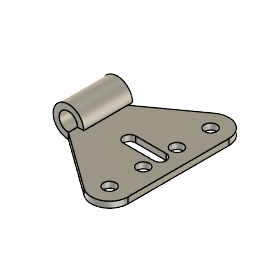
50 (Autodesk Fusion 360 design; units mm, degrees)
Autodesk Fusion 360 part; units mm, degrees
sketch "草图1" plane through (0, 0, 0) normal (0, 1, 0) x (1, 0, 0)
  line L0 (28, 3) -> (28, 5)
  line L1 (28, 5) -> (0, 5)
  arc A0 (0, 5) -> (5, 0) centre (0, 0) ccw
  line L2 (28, 3) -> (0, 3)
  arc A1 (0, 3) -> (3, 0) centre (0, 0) ccw
  line L3 (3, 0) -> (5, 0)
  line L4 (0, 3) -> (0, 5)
  dimension "d1" = 2
  dimension "d2" = 3
  dimension "d3" = 5
  dimension "d4" = 2
  dimension "d5" = 28
  constraint vertical L0
  constraint perpendicular L0 L1
  constraint tangent L1 A0
  constraint perpendicular L0 L2
  constraint tangent L2 A1
  constraint parallel L2 L3
  constraint coincident A0.centre A1.centre
  measures "d1" distance of L0.start L0.end
  measures "d2" radius of A1
  measures "d3" radius of A0
  measures "d4" distance of A0.end A1.end
  measures "d5" distance of L0.end L1.end
extrude "拉伸1" add sketch "草图1" along normal mid plane 16 contours A0 A1 L3 L4
extrude "拉伸2" add sketch "草图1" along normal mid plane 45 contours L0 L1 L2 L4
sketch "草图2" plane through (0, 0, -3) normal (0, 0, 1) x (-1, 0, 0)
  line L0 (-28, 22.5) -> (-28, -22.5)
  line L1 (-28, -22.5) -> (0, -22.5)
  line L2 (0, -22.5) -> (0, -8)
  line L3 (0, -8) -> (0, 8)
  line L4 (0, 8) -> (0, 22.5)
  line L5 (0, 22.5) -> (-28, 22.5)
  line L6 (0, -8) -> (-18.4849, -21.3625)
  arc A0 (-28, -16.5) -> (-18.4849, -21.3625) centre (-22, -16.5) ccw
  line L7 (-28, -16.5) -> (-28, 16.5)
  arc A1 (-18.4849, 21.3625) -> (-28, 16.5) centre (-22, 16.5) ccw
  line L8 (-18.4849, 21.3625) -> (0, 8)
  line L9 (0, 8) -> (0, -8)
  line L10 (10, 0) -> (-55, 0) construction
  circle A2 centre (-22, -16.5) radius 2
  circle A3 centre (-22, 16.5) radius 2
  line L11 (-22, -16.5) -> (-22, 16.5) construction
  circle A4 centre (-22, -5.5) radius 2
  circle A5 centre (-22, 5.5) radius 2
  circle A6 centre (-22, 16.5) radius 2
  line L12 (-12, 2) -> (-22, 2)
  arc A7 (-22, 2) -> (-22, -2) centre (-22, 0) ccw
  line L13 (-22, -2) -> (-12, -2)
  arc A8 (-12, -2) -> (-12, 2) centre (-12, 0) ccw
  dimension "d10" = 6
  dimension "d11" = 6
  dimension "d12" = 45
  dimension "d13" = 4
  dimension "d14" = 4
  dimension "d17" = 33
  dimension "d18" = 0
  dimension "d19" = 4
  dimension "d20" = 14
  constraint coincident L2.end L3.start
  constraint coincident L0 A0.start
  constraint tangent L6 A0
  constraint coincident L0 L7.end
  constraint tangent L7 A1
  constraint coincident L3.end L4.start
  constraint tangent A1 L8
  constraint tangent A0 L7
  constraint horizontal L10
  constraint symmetric A0.centre A1.centre L10
  constraint concentric A0 A2
  constraint concentric A1 A3
  constraint coincident A0.centre A2.centre
  constraint coincident A1.centre A3.centre
  constraint parallel L10 L12
  constraint coincident L11 A7.end
  constraint tangent L12 A7
  constraint tangent A7 L13
  constraint perpendicular L11 L13
  constraint tangent L13 A8
  constraint tangent L12 A8
  constraint collinear L10.end A7.centre A8.centre
  measures "d10" radius of A0
  measures "d11" radius of A1
  measures "d13" diameter of A2
  measures "d14" diameter of A3
  measures "d19" distance of L12 L13
extrude "拉伸3" cut sketch "草图2" against normal blind 11 contours L0 L5 A1 | L4 L5 A1 L8 | L0 L1 A0 | L1 L2 L6 A0 | A2 | A3 A6 | A4 | A5 | L12 A7 L13 A8
